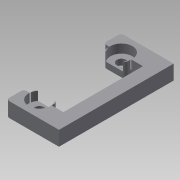
# Autodesk Inventor part: FixationCorona
Saved by Autodesk Inventor 2014 (Build 180170000, 170)
## iProperties
Created: 2013-11-13
Part Number: FixationCorona
Material: Générique
Document SubType Name: Modeling
Designer: Grégoire
Density: 1 g/cm^3
Appearance: Par défaut
Author: Grégoire
Autodesk Inventor part; units mm, degrees
ref_plane "YZ Plane" through (0, 0, 0) normal (1, 0, 0) x (0, 1, 0)
ref_plane "XZ Plane" through (0, 0, 0) normal (0, 1, 0) x (-1, 0, 0)
ref_plane "XY Plane" through (0, 0, 0) normal (0, 0, 1) x (1, 0, 0)
sketch "Esquisse1" plane through (0, 0, 0) normal (0, 0, 1) x (1, 0, 0)
  line L0 (-6, 11.6) -> (6, 11.6) construction
  line L1 (6, 11.6) -> (6, -11.6) construction
  line L2 (6, -11.6) -> (-6, -11.6) construction
  line L3 (-6, -11.6) -> (-6, 11.6) construction
  line L4 (-6, 11.6) -> (6, -11.6) construction
  line L5 (-6, -11.6) -> (6, 11.6) construction
  line L6 (-3.7, -11.6) -> (3.7, -11.6)
  line L7 (3.7, -11.6) -> (3.7, -13.6)
  line L8 (-3.7, -13.6) -> (-3.7, -11.6)
  line L9 (-5.75, -19.6) -> (6.25, -19.6)
  line L10 (-5.75, -13.6) -> (-5.75, -19.6)
  line L11 (5.75, -13.6) -> (3.7, -13.6)
  line L12 (-3.7, -13.6) -> (-5.75, -13.6)
  circle A0 centre (0, -14) radius 1.6
  line L13 (-3.7, -13.6) -> (0, -14) construction
  line L14 (0, -14) -> (3.7, -13.6) construction
  line L15 (-6, 0) -> (6, 0) construction
  line L16 (6, 0) -> (28.3304, 0) construction
  line L17 (7.75, 0) -> (7.75, -13.6)
  line L18 (12.25, -19.6) -> (12.25, 0)
  line L19 (5.75, -13.6) -> (7.75, -13.6)
  line L20 (6.25, -19.6) -> (12.25, -19.6)
  line L21 (6, -11.6) -> (6, 11.6) construction
  line L22 (6, 11.6) -> (-6, 11.6) construction
  line L23 (-6, 11.6) -> (-6, -11.6) construction
  line L24 (-6, -11.6) -> (6, 11.6) construction
  line L25 (-6, 11.6) -> (6, -11.6) construction
  line L26 (-3.7, 11.6) -> (3.7, 11.6)
  line L27 (3.7, 11.6) -> (3.7, 13.6)
  line L28 (-3.7, 13.6) -> (-3.7, 11.6)
  line L29 (-5.75, 19.6) -> (6.25, 19.6)
  line L30 (-5.75, 13.6) -> (-5.75, 19.6)
  line L31 (5.75, 13.6) -> (3.7, 13.6)
  line L32 (-3.7, 13.6) -> (-5.75, 13.6)
  circle A1 centre (0, 14) radius 1.6
  line L33 (-3.7, 13.6) -> (0, 14) construction
  line L34 (0, 14) -> (3.7, 13.6) construction
  line L35 (7.75, 0) -> (7.75, 13.6)
  line L36 (12.25, 19.6) -> (12.25, 0)
  line L37 (5.75, 13.6) -> (7.75, 13.6)
  line L38 (6.25, 19.6) -> (12.25, 19.6)
  point P0 (0, 0)
  point P1 (0, 0)
  point P2 (0, -11.6)
  point P3 (0, 11.6)
  dimension "d0" = 23.2
  dimension "d1" = 12
  dimension "d2" = 7.4
  dimension "d4" = 2
  dimension "d6" = 2.4
  dimension "d7" = 3.2
  dimension "d8" = 6
  dimension "d9" = 18
  dimension "d10" = 2
  dimension "d11" = 4.5
  constraints: 78 end point, 16 symmetric about line, 6 parallel, 5 midpoint, 4 horizontal, 3 equal length, 3 perpendicular, 3 point on line, 2 centre point, 2 collinear, 1 coincident, 1 other
  measures "d0" distance of L2.end L0.start
  measures "d1" distance of L0.start L0.end
  measures "d2" distance of L6.start L6.end
  measures "d4" distance of L6.end L7.end
  measures "d6" distance of point (0, -11.6) L13.end
  measures "d7" diameter of A0
  measures "d8" distance of L10.start L9.start
  measures "d9" distance between parallel lines of L10 L18
  measures "d10" distance of L11.start L17.end
  measures "d11" distance between parallel lines of L17 L18
extrude "Extrusion1" add sketch "Esquisse1" along normal blind 5
sketch "Esquisse2" plane through (0, 0, 5) normal (0, 0, 1) x (1, 0, 0)
  circle A0 centre (0, 14) radius 1.6 construction
  line L0 (12.25, -19.6) -> (12.25, 19.6) construction
  line L1 (3.7, -13.6) -> (3.7, -11.6) construction
  circle A1 centre (0, 14) radius 3.75
  line L2 (12.25, 0) -> (-17.9145, 0) construction
  circle A2 centre (0, -14) radius 3.75
  point P0 (0, 0)
  dimension "d14" = 7.5
  constraints: 2 centre point, 2 end point, 1 coincident, 1 midpoint, 1 perpendicular, 1 symmetric about line, 1 other
  measures "d14" diameter of A1
extrude "Extrusion2" cut sketch "Esquisse2" against normal blind 3
fillet "Congé1" radius 1 4 edges at (3.7, 11.6, 2.5) (-3.7, 11.6, 2.5) (3.7, -11.6, 2.5) (-3.7, -11.6, 2.5)
fillet "Congé2" radius 1 4 edges at (-5.75, 13.6, 2.5) (-5.75, 19.6, 2.5) (-5.75, -13.6, 2.5) (-5.75, -19.6, 2.5)
